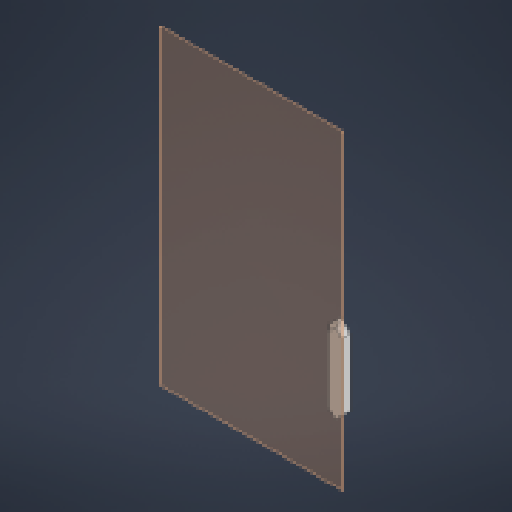
# Autodesk Inventor part: Spacer_1
Saved by Autodesk Inventor 2023.4 (Build 274418000, 418)
## iProperties
Created: 2025-10-22
Part Number: Spacer_1
Material: Generic
Document SubType Name: Modeling
Designer: Malthe Sennels
Density: 1 g/cm^3
Appearance: Default
Author: Malthe Sennels
Autodesk Inventor part; units mm, degrees
ref_plane "YZ Plane" through (0, 0, 0) normal (1, 0, 0) x (0, 1, 0)
ref_plane "XZ Plane" through (0, 0, 0) normal (0, 1, 0) x (-1, 0, 0)
ref_plane "XY Plane" through (0, 0, 0) normal (0, 0, 1) x (1, 0, 0)
ref_plane "Work Plane1" through (0, 0, 0) normal (0, 0, 1) x (1, 0, 0)
sketch "Sketch1" plane through (0, 0, 0) normal (0, 0, 1) x (1, 0, 0)
  line L0 (57, -68) -> (57, -18) projected
  line L1 (57, -18) -> (62, -13) projected
  line L2 (62, -73) -> (57, -68) projected
  line L3 (62, -73) -> (67, -68)
  line L4 (67, -68) -> (67, -18)
  line L5 (67, -18) -> (62, -13)
  line L6 (62.1414, -13.1414) -> (57.2, -18.0828)
  line L7 (57.2, -18.0828) -> (57.2, -67.9172)
  line L8 (57.2, -67.9172) -> (62.1414, -72.8586)
  point P0 (0, 0)
  dimension "d0" = 135
  dimension "d1" = 0.2
  dimension "d2" = 0.2
  dimension "d3" = 0.2
  dimension "d4" = 5
  constraints: 12 end point, 3 perpendicular, 2 point on line, 1 parallel
  measures "d0" angle of L4 L3
  measures "d1" distance between parallel lines of L0 L7
  measures "d2" distance between parallel lines of L2 L8
  measures "d3" distance between parallel lines of L1 L6
  measures "d4" distance from line of L4 L1.end
extrude "Extrusion1" add sketch "Sketch1" against normal blind 3.2 contours L8 L7 L6 L5 L4 L3
sketch "Sketch2" plane through (0, 0, -3.2) normal (0, 0, -1) x (-1, 0, 0)
  line L0 (-62.1414, -13.1414) -> (-67, -18) projected
  line L1 (-67, -18) -> (-67, -68) projected
  line L2 (-67, -68) -> (-62.1414, -72.8586) projected
  line L3 (-62.1414, -72.8586) -> (-57.2, -67.9172) projected
  line L4 (-57.2, -67.9172) -> (-57.2, -18.0828) projected
  line L5 (-57.2, -18.0828) -> (-62.1414, -13.1414) projected
  line L6 (-62.1414, -72.8586) -> (-57.2, -67.9172) projected
  line L7 (-62.1414, -72.8586) -> (-60.0201, -74.9799)
  line L8 (-62.1414, -72.8586) -> (-59.1414, -72.8586) construction
  line L9 (-60.0201, -74.9799) -> (-54.2, -69.1598)
  line L10 (-54.2, -69.1598) -> (-54.2, -16.8402)
  line L11 (-54.2, -16.8402) -> (-60.0201, -11.0201)
  line L12 (-62.1414, -13.1414) -> (-67, -18) projected
  line L13 (-60.0201, -11.0201) -> (-62.1414, -13.1414)
  point P0 (0, 0)
  dimension "d7" = 3
  dimension "d8" = 45
  dimension "d9" = 3
  dimension "d10" = 3
  constraints: 12 end point, 3 perpendicular, 1 equal length, 1 horizontal, 1 vertical
  measures "d7" distance of L2.end L7.end
  measures "d8" angle of L7 L8
  measures "d9" distance between parallel lines of L11 L5
  measures "d10" distance between parallel lines of L10 L4
extrude "Extrusion2" add sketch "Sketch2" along normal blind 3
sketch "Sketch3" plane through (0, 0, 0) normal (0, 0, 1) x (1, 0, 0)
  line L0 (67, -18) -> (62.1414, -13.1414) projected
  line L1 (62.1414, -13.1414) -> (57.2, -18.0828) projected
  line L2 (57.2, -18.0828) -> (57.2, -67.9172) projected
  line L3 (57.2, -67.9172) -> (62.1414, -72.8586) projected
  line L4 (62.1414, -72.8586) -> (67, -68) projected
  line L5 (67, -68) -> (67, -18) projected
  line L6 (60.0201, -11.0201) -> (62.1414, -13.1414) projected
  line L7 (54.2, -16.8402) -> (60.0201, -11.0201) projected
  line L8 (54.2, -69.1598) -> (54.2, -16.8402) projected
  line L9 (60.0201, -74.9799) -> (54.2, -69.1598) projected
  line L10 (62.1414, -72.8586) -> (60.0201, -74.9799) projected
  point P0 (0, 0)
extrude "Extrusion3" add sketch "Sketch3" along normal blind 2
ref_plane "Work Plane2" through (62.1414, -13.1414, 0) normal (1, 0, 0) x (0, 0, -1)
sketch "Sketch4" plane through (62.1414, -13.1414, 0) normal (1, 0, 0) x (0, 0, -1)
  line L0 (0, 0.1414) -> (0, 40.1414) projected
  line L1 (-30.4, 40.1414) -> (-30.4, 0.1414) projected
  line L2 (-30.4, 0.1414) -> (0, 0.1414) construction
  line L3 (-15.2, 0.1414) -> (-15.2, -64.0038) construction
  line L4 (-2, -4.8586) -> (6.2, -4.8586) projected
  line L5 (6.2, -54.8586) -> (-2, -54.8586) projected
  line L6 (-2, -54.8586) -> (-2, -4.8586) projected
  line L7 (-2, -4.8586) -> (-15.2, -4.8586)
  line L8 (-15.2, -4.8586) -> (-15.2, -54.8586)
  line L9 (-15.2, -54.8586) -> (-2, -54.8586)
  line L10 (-2, -54.8586) -> (-2, -4.8586)
  line L11 (-15.2, -11.8586) -> (-2, -11.8586)
  line L12 (-2, -11.8586) -> (-2, -47.8586)
  line L13 (-2, -47.8586) -> (-15.2, -47.8586)
  line L14 (-15.2, -47.8586) -> (-15.2, -11.8586)
  point P0 (0, 13.1414)
  point P1 (-2, -11.8586)
  dimension "d15" = 7
  dimension "d16" = 7
  constraints: 20 end point, 4 parallel, 4 point on line, 3 horizontal, 2 perpendicular, 1 midpoint, 1 vertical
  measures "d15" distance between parallel lines of L9 L13
  measures "d16" distance between parallel lines of L7 L11
extrude "Extrusion4" add sketch "Sketch4" along normal mid plane 6 contours L9 L8 L13 L6 | L11 L8 L7 L6
mirror "Mirror1" about plane through (62.1414, -61, 15.2) normal (0, 0, 1) of "Extrusion1", "Extrusion3", "Extrusion2", "Extrusion4"
fillet "Fillet1" radius 2 4 edges at (65.1414, -18, 15.2) (59.1414, -18, 15.2) (65.1414, -68, 15.2) (59.1414, -68, 15.2)
sketch "Sketch5" plane through (0, 0, 2) normal (0, 0, 1) x (1, 0, 0)
  line L0 (63, -53) -> (69, -53) projected
  line L1 (71, -51) -> (71, -45) projected
  arc A0 (69, -53) -> (71, -51) centre (69, -51) ccw projected
  arc A1 (71, -45) -> (69, -43) centre (69, -45) ccw projected
  line L2 (69, -43) -> (63, -43) projected
  line L3 (67, -18) -> (67, -68) projected
  line L4 (70.4142, -52.4142) -> (67, -55.8284)
  line L5 (67, -68) -> (67, -18) projected
  line L6 (70.4142, -43.5858) -> (67, -40.1716)
  point P0 (0, 0)
  constraints: 4 end point, 2 point on circle, 2 point on line, 2 tangent
extrude "Extrusion5" add sketch "Sketch5" against normal up to surface (8.2 mm away)
sketch "Sketch6" plane through (0, 0, 2) normal (0, 0, 1) x (1, 0, 0)
  line L0 (71, -51) -> (71, -45) projected
  circle A0 centre (66, -48) radius 1.5 construction
  line L1 (69, -49.7321) -> (66, -51.4641)
  line L2 (66, -51.4641) -> (63, -49.7321)
  line L3 (63, -49.7321) -> (63, -46.2679)
  line L4 (63, -46.2679) -> (66, -44.5359)
  line L5 (66, -44.5359) -> (69, -46.2679)
  line L6 (69, -46.2679) -> (69, -49.7321)
  point P0 (0, 0)
  dimension "d22" = 6
  constraints: 12 end point, 1 coincident, 13 other
  measures "d22" distance between parallel lines of L6 L3
extrude "Extrusion6" cut sketch "Sketch6" against normal blind 5.2
sketch "Sketch7" plane through (0, 0, -3.2) normal (0, 0, 1) x (1, 0, 0)
  line L0 (66, -44.5359) -> (69, -46.2679) projected
  line L1 (63, -46.2679) -> (66, -44.5359) projected
  line L2 (63, -49.7321) -> (63, -46.2679) projected
  line L3 (66, -51.4641) -> (63, -49.7321) projected
  line L4 (69, -49.7321) -> (66, -51.4641) projected
  line L5 (69, -46.2679) -> (69, -49.7321) projected
  circle A0 centre (66, -48) radius 1.5 construction
  circle A1 centre (66, -48) radius 1.75
  point P0 (0, 0)
  dimension "d25" = 3.5
  constraints: 1 centre point, 1 coincident
  measures "d25" diameter of A1
extrude "Extrusion7" cut sketch "Sketch7" against normal blind 5.2 contours A1
sketch "Sketch8" plane through (54.2, -69.1598, 28.4) normal (0, 0, -1) x (-1, 0, 0)
  line L0 (-4.9414, 8.1598) -> (-10.9414, 8.1598) projected
  line L1 (-10.9414, 8.1598) -> (-10.9414, 3.1598) projected
  arc A0 (-10.9414, 3.1598) -> (-8.9414, 1.1598) centre (-8.9414, 3.1598) ccw projected
  line L2 (-8.9414, 1.1598) -> (-6.9414, 1.1598) projected
  arc A1 (-6.9414, 1.1598) -> (-4.9414, 3.1598) centre (-6.9414, 3.1598) ccw projected
  line L3 (-4.9414, 3.1598) -> (-4.9414, 8.1598) projected
  line L4 (-10.9414, 49.1598) -> (-10.9414, 44.1598) projected
  line L5 (-10.9414, 44.1598) -> (-4.9414, 44.1598) projected
  line L6 (-4.9414, 44.1598) -> (-4.9414, 49.1598) projected
  arc A2 (-4.9414, 49.1598) -> (-6.9414, 51.1598) centre (-6.9414, 49.1598) ccw projected
  line L7 (-6.9414, 51.1598) -> (-8.9414, 51.1598) projected
  arc A3 (-8.9414, 51.1598) -> (-10.9414, 49.1598) centre (-8.9414, 49.1598) ccw projected
  line L8 (-8.9414, 1.1598) -> (-6.9414, 1.1598) projected
  arc A4 (-10.9414, 3.1598) -> (-8.9414, 1.1598) centre (-8.9414, 3.1598) ccw projected
  line L9 (-10.9414, 8.1598) -> (-10.9414, 3.1598) projected
  line L10 (-4.9414, 8.1598) -> (-10.9414, 8.1598) projected
  line L11 (-4.9414, 3.1598) -> (-4.9414, 8.1598) projected
  arc A5 (-6.9414, 1.1598) -> (-4.9414, 3.1598) centre (-6.9414, 3.1598) ccw projected
  line L12 (-4.9414, 44.1598) -> (-4.9414, 49.1598) projected
  line L13 (-10.9414, 44.1598) -> (-4.9414, 44.1598) projected
  line L14 (-10.9414, 49.1598) -> (-10.9414, 44.1598) projected
  arc A6 (-8.9414, 51.1598) -> (-10.9414, 49.1598) centre (-8.9414, 49.1598) ccw projected
  line L15 (-6.9414, 51.1598) -> (-8.9414, 51.1598) projected
  arc A7 (-4.9414, 49.1598) -> (-6.9414, 51.1598) centre (-6.9414, 49.1598) ccw projected
  line L16 (-12.8, 1.1598) -> (-12.8, 51.1598) projected
  line L17 (-5.8201, -5.8201) -> (-12.8, 1.1598) projected
  line L18 (0, 0) -> (-5.8201, -5.8201) projected
  line L19 (0, 52.3196) -> (0, 0) projected
  line L20 (-5.8201, 58.1397) -> (0, 52.3196) projected
  line L21 (-12.8, 51.1598) -> (-5.8201, 58.1397) projected
  line L22 (-10.9, 27.8918) -> (-7.9, 29.6239)
  line L23 (-7.9, 29.6239) -> (-4.9, 27.8918)
  line L24 (-4.9, 27.8918) -> (-4.9, 24.4277)
  line L25 (-4.9, 24.4277) -> (-7.9, 22.6957)
  line L26 (-7.9, 22.6957) -> (-10.9, 24.4277)
  line L27 (-10.9, 24.4277) -> (-10.9, 27.8918)
  line L28 (-7.8, 56.1598) -> (-2.8, 51.1598) projected
  line L29 (-7.9414, 56.0184) -> (-3, 51.077) projected
  line L30 (-3, 1.2426) -> (-7.9414, -3.6988) projected
  line L31 (-3, 51.077) -> (-3, 1.2426) projected
  line L32 (-3, 26.1598) -> (-12.8, 26.1598) construction
  line L33 (-7.9, 26.1598) -> (-7.9414, 44.1598) construction
  line L34 (-4.9276, 36.4277) -> (-7.9276, 34.6957)
  line L35 (-7.9276, 34.6957) -> (-10.9276, 36.4277)
  line L36 (-10.9276, 36.4277) -> (-10.9276, 39.8918)
  line L37 (-10.9276, 39.8918) -> (-7.9276, 41.6239)
  line L38 (-7.9276, 41.6239) -> (-4.9276, 39.8918)
  line L39 (-4.9276, 39.8918) -> (-4.9276, 36.4277)
  line L40 (-4.9276, 15.8918) -> (-7.9276, 17.6239)
  line L41 (-7.9276, 17.6239) -> (-10.9276, 15.8918)
  line L42 (-10.9276, 15.8918) -> (-10.9276, 12.4277)
  line L43 (-10.9276, 12.4277) -> (-7.9276, 10.6957)
  line L44 (-7.9276, 10.6957) -> (-4.9276, 12.4277)
  line L45 (-4.9276, 12.4277) -> (-4.9276, 15.8918)
  point P0 (54.2, 69.1598)
  point P1 (-7.8, -3.8402)
  point P2 (-7.9276, 38.1598)
  dimension "d28" = 6
  dimension "d29" = 6
  dimension "d30" = 12
  constraints: 40 end point, 6 symmetric about line, 5 midpoint, 3 parallel, 1 point on line, 27 other
  measures "d28" distance between parallel lines of L27 L24
  measures "d29" distance between parallel lines of L36 L39
  measures "d30" vertical distance of point (-7.928, 38.16) L33.start
extrude "Extrusion8" cut sketch "Sketch8" against normal blind 4 contours L22 L23 L24 L25 L26 L27 | L34 L35 L36 L37 L38 L39 | L45 L44 L43 L42 L41 L40
sketch "Sketch9" plane through (54.2, -69.1598, 32.4) normal (0, 0, -1) x (-1, 0, 0)
  line L0 (-7.9276, 41.6239) -> (-4.9276, 39.8918) projected
  line L1 (-10.9276, 39.8918) -> (-7.9276, 41.6239) projected
  line L2 (-10.9276, 36.4277) -> (-10.9276, 39.8918) projected
  line L3 (-7.9276, 34.6957) -> (-10.9276, 36.4277) projected
  line L4 (-4.9276, 36.4277) -> (-7.9276, 34.6957) projected
  line L5 (-4.9276, 39.8918) -> (-4.9276, 36.4277) projected
  line L6 (-7.9, 22.6957) -> (-10.9, 24.4277) projected
  line L7 (-4.9, 24.4277) -> (-7.9, 22.6957) projected
  line L8 (-4.9, 27.8918) -> (-4.9, 24.4277) projected
  line L9 (-7.9, 29.6239) -> (-4.9, 27.8918) projected
  line L10 (-10.9, 27.8918) -> (-7.9, 29.6239) projected
  line L11 (-10.9, 24.4277) -> (-10.9, 27.8918) projected
  line L12 (-4.9276, 15.8918) -> (-4.9276, 12.4277) projected
  line L13 (-7.9276, 17.6239) -> (-4.9276, 15.8918) projected
  line L14 (-10.9276, 15.8918) -> (-7.9276, 17.6239) projected
  line L15 (-10.9276, 12.4277) -> (-10.9276, 15.8918) projected
  line L16 (-7.9276, 10.6957) -> (-10.9276, 12.4277) projected
  line L17 (-4.9276, 12.4277) -> (-7.9276, 10.6957) projected
  line L18 (-7.9276, 41.6239) -> (-4.9276, 39.8918) projected
  line L19 (-7.9276, 41.6239) -> (-7.9276, 10.6957) construction
  circle A0 centre (-7.9276, 38.1598) radius 1.75
  circle A1 centre (-7.9276, 26.1598) radius 1.75
  circle A2 centre (-7.9276, 14.1598) radius 1.75
  line L20 (-6.4276, 40.7579) -> (-7.9276, 38.1598) construction
  line L21 (-7.9276, 14.1598) -> (-6.4276, 11.5617) construction
  point P0 (54.2, 69.1598)
  dimension "d33" = 3.5
  dimension "d34" = 3.5
  dimension "d35" = 3.5
  constraints: 6 end point, 3 centre point, 3 midpoint, 2 perpendicular, 2 point on line
  measures "d33" diameter of A0
  measures "d34" diameter of A1
  measures "d35" diameter of A2
extrude "Extrusion9" cut sketch "Sketch9" against normal blind 12.5 contours A0 | A1 | A2
sketch "Sketch11" plane through (65.1414, -13.1414, 0) normal (1, 0, 0) x (0, 0, -1)
  line L0 (-2, -47.8586) -> (-28.4, -47.8586) projected
  line L1 (-15.2, -47.8586) -> (-15.2, -11.8586) construction
  line L2 (-2, -11.8586) -> (-28.4, -11.8586) projected
  line L3 (-12.2, -47.8586) -> (-18.2, -47.8586)
  line L4 (-18.2, -47.8586) -> (-18.2, -11.8586)
  line L5 (-18.2, -11.8586) -> (-12.2, -11.8586)
  line L6 (-12.2, -11.8586) -> (-12.2, -47.8586)
  line L7 (-12.2, -47.8586) -> (-18.2, -11.8586) construction
  line L8 (-18.2, -47.8586) -> (-12.2, -11.8586) construction
  point P0 (0, 13.1414)
  point P1 (-15.2, -29.8586)
  dimension "d40" = 6
  constraints: 14 end point, 5 midpoint, 2 parallel, 1 horizontal, 1 perpendicular, 1 point on line
  measures "d40" distance between parallel lines of L6 L4
extrude "Extrusion10" add sketch "Sketch11" against normal up to surface (6 mm away)
fillet "Fillet2" radius 2 8 edges at (59.1414, -43, 12.2) (59.1414, -43, 18.2) (65.1414, -43, 18.2) (65.1414, -43, 12.2) (62.1414, -61, 18.2) (62.1414, -61, 12.2) (62.1414, -25, 18.2) (62.1414, -25, 12.2)
body "Solid1"
